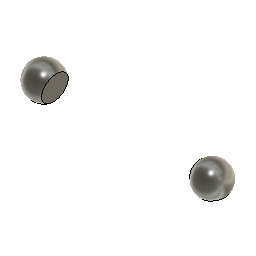
final arm part1 dr robot (Autodesk Fusion 360 design; units mm, degrees)
part number: 2026-03-12-10-30-56-626
Autodesk Fusion 360 part; units mm, degrees
sketch "Sketch1" plane through (0, 0, 0) normal (0, 1, 0) x (1, 0, 0)
  line L0 (27.3752, -25.2661) -> (26.7473, -20.2823) construction
  line L1 (22.4792, -21.28) -> (26.7473, -20.2823)
  point P0 (27.3752, -25.2661)
  point P1 (26.7473, -20.2823)
  point P2 (56.2579, -25.2661)
  point P3 (56, -21)
  point P4 (22.4792, -21.28)
  point P5 (26.7473, -20.2823)
  constraint coincident P0 L0.start
  constraint coincident P5 P1
  constraint coincident P4 L1.start
sphere "SpherePrimitive1" add diameter 6.8 placed x (1, 0, 0) y (0, 0, -1) z (0, 1, 0) at (25.0366, 0, 22.7742) makes body 1
move_body "Move1" bodies 1 to x (1, 0, 0) y (0, 1, 0) z (0, 0, 1) at (0, 0, 1)
ref_plane "WorkPlane1" through (27.0612, 0, 22.7742) normal (0.992157, 0, -0.124996) x (-0.124996, 0, -0.992157)
ref_plane "WorkPlane2" through (30.0377, 0, 22.3992) normal (0.992157, 0, -0.124996) x (-0.124996, 0, -0.992157)
sketch "Sketch4" plane through (26.7905, 0, -3.3752) normal (0.992157, 0, -0.124996) x (-0.124996, 0, -0.992157)
box "BoxPrimitive1" cut length 7.157 width 8.299 height -3 placed x (0, -1, 0) y (-0.124996, 0, -0.992157) z (0.992157, 0, -0.124996) at (30.6029, 3.5, 26.8856) bodies 1
ref_plane "WorkPlane3" through (24.6132, 0, 20.7812) normal (0.227632, 0, 0.973747) x (0.973747, 0, -0.227632)
ref_plane "WorkPlane4" through (24.158, 0, 18.8337) normal (0.227632, 0, 0.973747) x (0.973747, 0, -0.227632)
sketch "Sketch5" plane through (5.4264, 0, 23.2125) normal (0.227632, 0, 0.973747) x (0.973747, 0, -0.227632)
box "BoxPrimitive2" cut length 7.629 width 8.441 height 2.5 placed x (0, 1, 0) y (-0.973747, 0, 0.227632) z (0.227632, 0, 0.973747) at (27.8226, -3.629, 17.977) bodies 1
move_body "Move2" bodies 1 to x (1, 0, 0) y (0, 1, 0) z (0, 0, 1) at (0, 0, -0.5)
sketch "Sketch8" plane through (0, 0, 0) normal (0, 1, 0) x (1, 0, 0)
  line L0 (23, -12) -> (26, -13) construction
  line L1 (22.3127, -12.4707) -> (26.9903, -14.0299) construction
  point P0 (23, -12)
  point P1 (26, -13)
  point P2 (26.9903, -14.0299)
  point P3 (22.3127, -12.4707)
  constraint coincident P0 L0.start
  constraint coincident P1 L0.end
  constraint coincident P3 L1.start
  constraint coincident P2 L1.end
  constraint parallel L0 L1
ref_plane "WorkPlane5" through (24.6515, 0, 13.2503) normal (-0.316228, 0, 0.948683) x (0.948683, 0, 0.316228)
ref_plane "WorkPlane6" through (24.8614, 0, 12.6205) normal (-0.316228, 0, 0.948683) x (0.948683, 0, 0.316228)
sketch "Sketch9" plane through (-1.5099, 0, 4.5298) normal (-0.316228, 0, 0.948683) x (0.948683, 0, 0.316228)
  circle A0 centre (27.5765, 0) radius 2.4653
  point P0 (25.1112, 0)
  point P1 (30.0418, 0)
  constraint coincident P1 A0
  constraint coincident P0 A0
sketch "Sketch10" plane through (-1.3, 0, 3.9) normal (-0.316228, 0, 0.948683) x (0.948683, 0, 0.316228)
  circle A0 centre (27.1956, 0) radius 1.5811
  point P0 (28.7767, 0)
  point P1 (25.6144, 0)
  constraint coincident P1 A0
  constraint coincident P0 A0
sketch "Sketch11" plane through (0, 0, 0) normal (0, 1, 0) x (1, 0, 0)
  circle A0 through (22.2327, -21.3511, 0) (25.5812, -20.5684, 1.9854) (25.5812, -20.5684, -1.9854)
  circle A1 through (26.8227, -20.3812, 0) (27.319, -24.3207, 2.2925) (27.319, -24.3207, -2.2925)
  circle A2 through (22.3127, -12.4707, 0) (25.8209, -13.6401, 2.135) (25.8209, -13.6401, -2.135)
  circle A3 through (23, -12, 0) (25.25, -12.75, 1.3693) (25.25, -12.75, -1.3693)
  spline S0 degree 5 poles (22.246, -21.348, -0.2492) (22.2348, -21.0385, -0.2563) (22.2135, -20.4295, -0.2695) (22.1843, -19.546, -0.2866) (22.1512, -18.4293, -0.3038) (22.1203, -17.1434, -0.3153) (22.101, -15.9814, -0.3154) (22.0951, -14.961, -0.3026) (22.1044, -14.1011, -0.2752) (22.1304, -13.418, -0.2316) (22.1736, -12.9165, -0.1713) (22.2214, -12.6552, -0.1104) (22.2643, -12.5342, -0.0578) (22.2961, -12.4864, -0.0198) (22.3127, -12.4707, 0) knots 0 0 0 0 0 0 0.1 0.2 0.3 0.4 0.5 0.6 0.7 0.8 0.9 1 1 1 1 1 1
  spline S1 degree 5 poles (26.6873, -20.3098, -0.218) (26.7411, -20.2601, -0.2256) (26.8444, -20.152, -0.2391) (26.9863, -19.9642, -0.2546) (27.1492, -19.6619, -0.2659) (27.308, -19.1968, -0.264) (27.4206, -18.6463, -0.2465) (27.4861, -18.0174, -0.2149) (27.5048, -17.3252, -0.1721) (27.4784, -16.5954, -0.1232) (27.4096, -15.8598, -0.0743) (27.3017, -15.1532, -0.0323) (27.158, -14.5096, -0.0037) (26.9815, -13.9588, 0.0057) (26.7749, -13.5224, -0.0084) (26.5404, -13.2101, -0.0477) (26.3317, -13.0616, -0.0998) (26.1636, -13.0068, -0.1503) (26.0466, -12.9952, -0.1891) (25.9867, -12.9956, -0.2097) knots 0 0 0 0 0 0 0.06666667 0.13333333 0.2 0.26666667 0.33333333 0.4 0.46666667 0.53333333 0.6 0.66666667 0.73333333 0.8 0.86666667 0.93333333 1 1 1 1 1 1
  spline S2 degree 5 poles (22.3127, -12.4707) (22.3402, -12.4518) (22.3952, -12.4142) (22.4776, -12.3577) (22.5876, -12.2824) (22.7251, -12.1883) (22.835, -12.113) (22.9175, -12.0565) (22.9725, -12.0188) (23, -12) knots 0 0 0 0 0 0 0.2 0.4 0.6 0.8 1 1 1 1 1 1
  point P0 (22.1208, -13.7489)
  point P1 (27.4669, -18.1085)
  point P2 (26.9903, -14.0299)
sketch "Sketch12" plane through (0, 0, 0) normal (0, 1, 0) x (1, 0, 0)
  line L0 (56, -21) -> (56.2579, -25.2661) construction
  line L1 (57, -20) -> (61, -21) construction
  point P0 (57, -20)
  point P1 (61, -21)
  point P2 (56, -21)
  point P3 (56.2579, -25.2661)
  constraint coincident P2 L0.start
  constraint coincident P3 L0.end
  constraint coincident P0 L1.start
  constraint coincident P1 L1.end
ref_plane "WorkPlane7" through (56.1289, 0, 23.1331) normal (-0.998178, 0, 0.060338) x (0.060338, 0, 0.998178)
ref_plane "WorkPlane8" through (59, 0, 20.5) normal (-0.242536, 0, 0.970143) x (0.970143, 0, 0.242536)
ref_plane "WorkPlane9" through (54.1326, 0, 23.2537) normal (-0.998178, 0, 0.060338) x (0.060338, 0, 0.998178)
ref_plane "WorkPlane10" through (59.4851, 0, 18.5597) normal (-0.242536, 0, 0.970143) x (0.970143, 0, 0.242536)
sphere "SpherePrimitive2" add diameter 6.5 placed x (1, 0, 0) y (0, 0, -1) z (0, 1, 0) at (58.7124, 0, 23.0269) separate body makes body 2
move_body "Move3" bodies 2 to x (1, 0, 0) y (0, 1, 0) z (0, 0, 1) at (0, 0, 0.5)
move_body "Move4" bodies 2 to x (1, 0, 0) y (0, 1, 0) z (0, 0, 1) at (0, 0, -0.5)
sketch "Sketch15" plane through (52.535, 0, -3.1756) normal (-0.998178, 0, 0.060338) x (0.060338, 0, 0.998178)
box "BoxPrimitive3" cut length 7.285 width 9.713 height -2 placed x (0, 1, 0) y (-0.060338, 0, -0.998178) z (-0.998178, 0, 0.060338) at (54.3573, -3.5386, 26.9706) bodies 2
sketch "Sketch16" plane through (-0.8679, 0, 3.4715) normal (-0.242536, 0, 0.970143) x (0.970143, 0, 0.242536)
box "BoxPrimitive4" cut length 8 width 10 height 2 placed x (0, -1, 0) y (0.970143, 0, 0.242536) z (-0.242536, 0, 0.970143) at (54.4303, 4, 17.296) bodies 2
